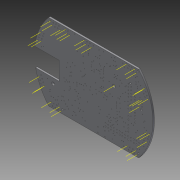
# Autodesk Inventor part: beep_main_new
Saved by Autodesk Inventor 2014 (Build 180170000, 170)
## iProperties
Created: 2013-08-27
Part Number: beep_main_new
Material: Generisch
Document SubType Name: Modeling
Designer: Felix
Density: 1 g/cm^3
Appearance: Vorgabe
Author: Felix
Autodesk Inventor part; units mm, degrees
ref_plane "YZ Plane" through (0, 0, 0) normal (1, 0, 0) x (0, 1, 0)
ref_plane "XZ Plane" through (0, 0, 0) normal (0, 1, 0) x (-1, 0, 0)
ref_plane "XY Plane" through (0, 0, 0) normal (0, 0, 1) x (1, 0, 0)
sketch "Skizze2" plane through (0, 0, 0) normal (0, 1, 0) x (-1, 0, 0)
  circle A0 centre (77.705, 71.07) radius 0.75
  circle A1 centre (17.77, 43.405) radius 0.75
  circle A2 centre (17.67, 60.315) radius 0.75
  circle A3 centre (7.87, 44.425) radius 0.75
  circle A4 centre (11.055, 72.63) radius 0.75
  circle A5 centre (10.255, 9.23) radius 0.75
  arc A6 (10.3, 74.8) -> (10.3, 5.7) centre (50.45, 40.25) ccw
  circle A7 centre (60.675, 71.27) radius 0.75
  circle A8 centre (78.855, 9.13) radius 0.75
  circle A9 centre (91.045, 71.07) radius 0.75
  circle A10 centre (32.7, 50.6) radius 1.4
  circle A11 centre (87.3, 25.1) radius 1.4
  arc A12 (91.4, 5.7) -> (103.1, 29.6999) centre (50.8775, 40.3065) ccw
  arc A13 (103.8, 46.0999) -> (91.4, 74.8) centre (50.8494, 40.2512) ccw
  line L0 (81.9, 29.6999) -> (103.1, 29.6999)
  line L1 (81.9, 46.0999) -> (81.9, 29.6999)
  line L2 (103.8, 46.0999) -> (81.9, 46.0999)
  line L3 (10.3, 5.7) -> (91.4, 5.7)
  line L4 (10.3, 74.8) -> (91.4, 74.8)
  circle A14 centre (32.9, 25.7) radius 0.254
  circle A15 centre (41.7, 37.3) radius 0.254
  circle A16 centre (44, 39.8) radius 0.254
  circle A17 centre (42, 14.1) radius 0.254
  circle A18 centre (52.4, 59.6) radius 0.254
  circle A19 centre (52.9, 55.5) radius 0.254
  circle A20 centre (52.9, 57) radius 0.254
  circle A21 centre (55.6, 64.7) radius 0.254
  circle A22 centre (54.6, 67.8) radius 0.254
  circle A23 centre (73.4, 19.4) radius 0.254
  circle A24 centre (78.1, 19.4) radius 0.254
  circle A25 centre (77.4, 16.7) radius 0.254
  circle A26 centre (70.2, 16.8) radius 0.254
  circle A27 centre (77.3, 24.7) radius 0.254
  circle A28 centre (72.9, 27.3) radius 0.254
  circle A29 centre (22.25, 50.95) radius 0.254
  circle A30 centre (30.1, 38) radius 0.254
  circle A31 centre (31.9, 59.9) radius 0.254
  circle A32 centre (27.7, 33) radius 0.254
  circle A33 centre (28.8, 43.2) radius 0.254
  circle A34 centre (30.3, 34.6) radius 0.254
  circle A35 centre (34, 41.7) radius 0.254
  circle A36 centre (32.3, 57.4) radius 0.254
  circle A37 centre (70.6, 42.4) radius 0.254
  circle A38 centre (24.5, 72.5) radius 0.254
  circle A39 centre (71.1, 39.3) radius 0.254
  circle A40 centre (11.2, 60.8) radius 0.254
  circle A41 centre (22.2, 27.1) radius 0.254
  circle A42 centre (72.3, 38.7) radius 0.254
  circle A43 centre (38.7, 23.6) radius 0.254
  circle A44 centre (76, 14.9) radius 0.254
  circle A45 centre (34, 19.5) radius 0.254
  circle A46 centre (75.2, 44) radius 0.254
  circle A47 centre (76.7, 10.1) radius 0.254
  circle A48 centre (10.5, 64.9) radius 0.254
  circle A49 centre (4.7, 37.2) radius 0.254
  circle A50 centre (92.4, 26.6) radius 0.254
  circle A51 centre (62.5, 17.2) radius 0.254
  circle A52 centre (82.8, 17.4) radius 0.254
  circle A53 centre (67.8, 12.5) radius 0.254
  circle A54 centre (37.3, 21) radius 0.254
  circle A55 centre (82.7, 11.6) radius 0.254
  circle A56 centre (8.4, 63) radius 0.254
  circle A57 centre (30, 65.2) radius 0.254
  circle A58 centre (43.5, 43.4) radius 0.254
  circle A59 centre (5.7, 35.9) radius 0.254
  circle A60 centre (9.5, 12.8) radius 0.254
  circle A61 centre (36.7, 23.3) radius 0.254
  circle A62 centre (64.6, 17.4) radius 0.254
  circle A63 centre (3.3, 30.6) radius 0.254
  circle A64 centre (69.1, 12.5) radius 0.254
  circle A65 centre (90.2, 17.7) radius 0.254
  circle A66 centre (13.1, 67.2) radius 0.254
  circle A67 centre (11.7, 68.6) radius 0.254
  circle A68 centre (31.4, 66.7) radius 0.254
  circle A69 centre (43.6, 44.9) radius 0.254
  circle A70 centre (11.5, 12.1) radius 0.254
  circle A71 centre (70, 9) radius 0.254
  circle A72 centre (35.2, 22.6) radius 0.254
  circle A73 centre (90.1, 19.2) radius 0.254
  circle A74 centre (63.5, 15.5) radius 0.254
  circle A75 centre (14.7, 68.1) radius 0.254
  circle A76 centre (30.06, 67.74) radius 0.254
  circle A77 centre (42, 45) radius 0.254
  circle A78 centre (57.4, 38.4) radius 0.254
  circle A79 centre (37, 26.4) radius 0.254
  circle A80 centre (31.4, 25.7) radius 0.254
  circle A81 centre (63.5, 21.7) radius 0.254
  circle A82 centre (11.2, 59.3) radius 0.254
  circle A83 centre (23.7, 27.1) radius 0.254
  circle A84 centre (64.7, 24.4) radius 0.254
  circle A85 centre (35.6, 24.7) radius 0.254
  circle A86 centre (30.6, 23.7) radius 0.254
  circle A87 centre (65.5, 26.3) radius 0.254
  circle A88 centre (66.6, 29.3) radius 0.254
  circle A89 centre (79.7, 15.9) radius 0.254
  circle A90 centre (67.7, 30.3) radius 0.254
  circle A91 centre (97.8, 48.7) radius 0.254
  circle A92 centre (76.6, 32) radius 0.254
  circle A93 centre (74.1, 33.1) radius 0.254
  circle A94 centre (41.9, 55.5) radius 0.254
  circle A95 centre (77.5, 34.5) radius 0.254
  circle A96 centre (32.9, 70.3) radius 0.254
  circle A97 centre (26.85, 36.1) radius 0.254
  circle A98 centre (31.7, 12.5) radius 0.254
  circle A99 centre (12.6, 63.9) radius 0.254
  circle A100 centre (67.7, 48.9) radius 0.254
  circle A101 centre (95.9, 49.8) radius 0.254
  circle A102 centre (62, 37.1) radius 0.254
  circle A103 centre (62.9, 26.4) radius 0.254
  circle A104 centre (62.4, 47.4) radius 0.254
  circle A105 centre (73.5, 12.3) radius 0.254
  circle A106 centre (48.4, 36.7) radius 0.254
  circle A107 centre (68.9, 35.1) radius 0.254
  circle A108 centre (44.6, 51) radius 0.254
  circle A109 centre (59.5, 34.2) radius 0.254
  circle A110 centre (39.1, 36.7) radius 0.254
  circle A111 centre (54.2, 36.7) radius 0.254
  circle A112 centre (51.1, 72.8) radius 0.254
  circle A113 centre (31.8, 73.1) radius 0.254
  circle A114 centre (49, 45) radius 0.254
  circle A115 centre (42.2, 49.9) radius 0.254
  circle A116 centre (66.8, 10.8) radius 0.254
  circle A117 centre (85.4, 13.4) radius 0.254
  circle A118 centre (21.8, 20.7) radius 0.254
  circle A119 centre (30.2, 36.3) radius 0.254
  circle A120 centre (41.8, 57.1) radius 0.254
  circle A121 centre (58.5, 10.5) radius 0.254
  circle A122 centre (53.7, 39.4) radius 0.254
  circle A123 centre (52, 34.2) radius 0.254
  circle A124 centre (56.4, 26.4) radius 0.3
  circle A125 centre (61.1, 11.6) radius 0.254
  circle A126 centre (26.9, 58) radius 0.254
  circle A127 centre (6.5, 19.3) radius 0.254
  circle A128 centre (17.1, 34.8) radius 0.254
  circle A129 centre (5.7, 26.7) radius 0.254
  circle A130 centre (5.6, 16.8) radius 0.254
  circle A131 centre (34, 8.5) radius 0.254
  circle A132 centre (41.8, 58.5) radius 0.254
  circle A133 centre (45.1, 53.9) radius 0.254
  circle A134 centre (50.3, 54.3) radius 0.254
  circle A135 centre (67.9, 73.5) radius 0.254
  circle A136 centre (47.2, 65.3) radius 0.254
  circle A137 centre (46, 72.1) radius 0.254
  circle A138 centre (41, 61.6) radius 0.3
  circle A139 centre (42, 72.7) radius 0.254
  circle A140 centre (32.9, 66.6) radius 0.254
  circle A141 centre (44.9, 43.2) radius 0.254
  circle A142 centre (29.6, 29.9) radius 0.254
  circle A143 centre (16.7, 29.4) radius 0.254
  circle A144 centre (12.7, 24.2) radius 0.254
  circle A145 centre (65.9, 35.5) radius 0.254
  circle A146 centre (61.3, 43.4) radius 0.254
  circle A147 centre (72.1, 30.3) radius 0.254
  circle A148 centre (59, 51) radius 0.254
  circle A149 centre (58.4, 46.9) radius 0.254
  circle A150 centre (79.4, 19.3) radius 0.254
  circle A151 centre (65.9, 36.9) radius 0.254
  circle A152 centre (45.2, 68.1) radius 0.254
  circle A153 centre (34.6, 72) radius 0.254
  circle A154 centre (29.2, 60.5) radius 0.254
  circle A155 centre (36.7, 64) radius 0.254
  circle A156 centre (44.5, 60.4) radius 0.254
  circle A157 centre (12.6, 62.1) radius 0.254
  circle A158 centre (38.9, 64.9) radius 0.254
  circle A159 centre (22.4, 55.2) radius 0.254
  circle A160 centre (15.1, 28.8) radius 0.254
  circle A161 centre (45.6, 61.4) radius 0.254
  circle A162 centre (45.6, 65.5) radius 0.254
  circle A163 centre (25.4, 56.5) radius 0.254
  circle A164 centre (35.5, 64.8) radius 0.254
  circle A165 centre (29.3, 22.4) radius 0.254
  circle A166 centre (25.4, 11.6) radius 0.254
  circle A167 centre (58.5, 39.5) radius 0.3
  circle A168 centre (45.3, 55.9) radius 0.254
  circle A169 centre (64.5, 28.9) radius 0.254
  circle A170 centre (86.9, 14.5) radius 0.254
  circle A171 centre (46.7, 55.9) radius 0.254
  circle A172 centre (71.9, 41.7) radius 0.254
  circle A173 centre (48.2, 55.8) radius 0.254
  circle A174 centre (70, 50.1) radius 0.254
  circle A175 centre (71.8, 46.1) radius 0.254
  circle A176 centre (50.8, 61.1) radius 0.254
  circle A177 centre (59.9, 37.2) radius 0.254
  circle A178 centre (6.8, 41.4) radius 0.254
  circle A179 centre (11.3, 26.4) radius 0.254
  circle A180 centre (55.7, 66.7) radius 0.254
  circle A181 centre (45.8, 22.8) radius 0.254
  circle A182 centre (44.9, 26) radius 0.254
  circle A183 centre (72.5, 33.9) radius 0.254
  circle A184 centre (34.6, 31.6) radius 0.254
  circle A185 centre (23.5, 23.3) radius 0.254
  circle A186 centre (21.5, 56.3) radius 0.254
  circle A187 centre (9.1, 53.3) radius 0.254
  circle A188 centre (74.2, 47.9) radius 0.254
  circle A189 centre (75.5, 33.9) radius 0.254
  circle A190 centre (60.3, 17.1) radius 0.254
  circle A191 centre (35.9, 20.5) radius 0.254
  circle A192 centre (32.7, 20.5) radius 0.254
  circle A193 centre (89.105, 14.395) radius 0.254
  circle A194 centre (83.6, 14.3) radius 0.254
  circle A195 centre (74.7, 13.7) radius 0.254
  circle A196 centre (23.9, 8) radius 0.254
  circle A197 centre (23.9, 11.6) radius 0.254
  circle A198 centre (5.2, 31.8) radius 0.254
  circle A199 centre (10.4, 20.5) radius 0.254
  circle A200 centre (23.03, 70.23) radius 0.254
  circle A201 centre (41.7, 53) radius 0.254
  circle A202 centre (43.2, 51.5) radius 0.254
  circle A203 centre (44.1, 57.8) radius 0.254
  circle A204 centre (31.4, 70.3) radius 0.254
  circle A205 centre (40.4, 42.8) radius 0.254
  circle A206 centre (22.7, 43.5) radius 0.254
  circle A207 centre (19.9, 45) radius 0.254
  circle A208 centre (58.2, 64.5) radius 0.254
  circle A209 centre (65.6, 61.3) radius 0.254
  circle A210 centre (55.6, 63.3) radius 0.254
  circle A211 centre (46.2, 27.8) radius 0.254
  circle A212 centre (61, 69.2) radius 0.254
  circle A213 centre (50.4, 52.8) radius 0.254
  circle A214 centre (52.5, 52.8) radius 0.254
  circle A215 centre (41.8, 60) radius 0.254
  circle A216 centre (48.8, 39.9) radius 0.254
  circle A217 centre (45.9, 39.8) radius 0.254
  circle A218 centre (30.1, 39.4) radius 0.254
  circle A219 centre (37.1, 13.3) radius 0.254
  circle A220 centre (33.2, 13.3) radius 0.254
  circle A221 centre (76.305, 72.87) radius 0.4064
  circle A222 centre (75.035, 70.33) radius 0.4064
  circle A223 centre (73.765, 72.87) radius 0.4064
  circle A224 centre (72.495, 70.33) radius 0.4064
  circle A225 centre (60.3, 44.5) radius 0.254
  circle A226 centre (19.57, 42.005) radius 0.4064
  circle A227 centre (17.03, 40.735) radius 0.4064
  circle A228 centre (19.57, 39.465) radius 0.4064
  circle A229 centre (17.03, 38.195) radius 0.4064
  circle A230 centre (65.9, 33.9) radius 0.254
  circle A231 centre (19.47, 58.915) radius 0.4064
  circle A232 centre (16.93, 57.645) radius 0.4064
  circle A233 centre (19.47, 56.375) radius 0.4064
  circle A234 centre (16.93, 55.105) radius 0.4064
  circle A235 centre (19.47, 53.835) radius 0.4064
  circle A236 centre (16.93, 52.565) radius 0.4064
  circle A237 centre (19.47, 51.295) radius 0.4064
  circle A238 centre (16.93, 50.025) radius 0.4064
  circle A239 centre (19.47, 48.755) radius 0.4064
  circle A240 centre (16.93, 47.485) radius 0.4064
  circle A241 centre (71.9, 28.8) radius 0.254
  circle A242 centre (9.67, 45.825) radius 0.4064
  circle A243 centre (7.13, 47.095) radius 0.4064
  circle A244 centre (9.67, 48.365) radius 0.4064
  circle A245 centre (7.13, 49.635) radius 0.4064
  circle A246 centre (9.67, 50.905) radius 0.4064
  circle A247 centre (7.13, 52.175) radius 0.4064
  circle A248 centre (63.4, 37) radius 0.254
  circle A249 centre (12.455, 70.83) radius 0.4064
  circle A250 centre (13.725, 73.37) radius 0.4064
  circle A251 centre (14.995, 70.83) radius 0.4064
  circle A252 centre (16.265, 73.37) radius 0.4064
  circle A253 centre (17.535, 70.83) radius 0.4064
  circle A254 centre (18.805, 73.37) radius 0.4064
  circle A255 centre (20.075, 70.83) radius 0.4064
  circle A256 centre (21.345, 73.37) radius 0.4064
  circle A257 centre (59.2, 45.4) radius 0.254
  circle A258 centre (11.655, 7.43) radius 0.4064
  circle A259 centre (12.925, 9.97) radius 0.4064
  circle A260 centre (14.195, 7.43) radius 0.4064
  circle A261 centre (15.465, 9.97) radius 0.4064
  circle A262 centre (16.735, 7.43) radius 0.4064
  circle A263 centre (18.005, 9.97) radius 0.4064
  circle A264 centre (19.275, 7.43) radius 0.4064
  circle A265 centre (20.545, 9.97) radius 0.4064
  circle A266 centre (67.5, 21.8) radius 0.254
  circle A267 centre (4.9078, 62.6827) radius 0.4064
  circle A268 centre (6.7307, 60.5053) radius 0.4064
  circle A269 centre (3.895, 60.3534) radius 0.4064
  circle A270 centre (5.7179, 58.1759) radius 0.4064
  circle A271 centre (2.8821, 58.0241) radius 0.4064
  circle A272 centre (4.705, 55.8466) radius 0.4064
  circle A273 centre (1.8693, 55.6947) radius 0.4064
  circle A274 centre (3.6922, 53.5173) radius 0.4064
  circle A275 centre (0.3852, 29.2123) radius 0.4064
  circle A276 centre (3.1969, 28.8139) radius 0.4064
  circle A277 centre (1.1912, 26.8036) radius 0.4064
  circle A278 centre (4.0029, 26.4052) radius 0.4064
  circle A279 centre (1.9971, 24.3948) radius 0.4064
  circle A280 centre (4.8088, 23.9964) radius 0.4064
  circle A281 centre (2.8031, 21.9861) radius 0.4064
  circle A282 centre (5.6148, 21.5877) radius 0.4064
  circle A283 centre (59.275, 73.07) radius 0.4064
  circle A284 centre (58.005, 70.53) radius 0.4064
  circle A285 centre (56.735, 73.07) radius 0.4064
  circle A286 centre (55.465, 70.53) radius 0.4064
  circle A287 centre (54.195, 73.07) radius 0.4064
  circle A288 centre (30, 57.6) radius 0.254
  circle A289 centre (24.5, 48.9) radius 0.254
  circle A290 centre (80.255, 7.33) radius 0.4064
  circle A291 centre (81.525, 9.87) radius 0.4064
  circle A292 centre (82.795, 7.33) radius 0.4064
  circle A293 centre (84.065, 9.87) radius 0.4064
  circle A294 centre (85.335, 7.33) radius 0.4064
  circle A295 centre (86.605, 9.87) radius 0.4064
  circle A296 centre (87.875, 7.33) radius 0.4064
  circle A297 centre (89.145, 9.87) radius 0.4064
  circle A298 centre (30.9, 58.9) radius 0.254
  circle A299 centre (89.645, 72.87) radius 0.4064
  circle A300 centre (88.375, 70.33) radius 0.4064
  circle A301 centre (87.105, 72.87) radius 0.4064
  circle A302 centre (85.835, 70.33) radius 0.4064
  circle A303 centre (84.565, 72.87) radius 0.4064
  circle A304 centre (83.295, 70.33) radius 0.4064
  circle A305 centre (82.025, 72.87) radius 0.4064
  circle A306 centre (80.755, 70.33) radius 0.4064
  circle A307 centre (26.6, 45.4) radius 0.254
  circle A308 centre (97.1044, 17.2038) radius 0.4064
  circle A309 centre (95.2288, 19.3361) radius 0.4064
  circle A310 centre (98.06, 19.5572) radius 0.4064
  circle A311 centre (96.1844, 21.6895) radius 0.4064
  circle A312 centre (99.0156, 21.9105) radius 0.4064
  circle A313 centre (97.14, 24.0428) radius 0.4064
  circle A314 centre (99.9712, 24.2639) radius 0.4064
  circle A315 centre (98.0956, 26.3962) radius 0.4064
  circle A316 centre (101.1281, 52.2968) radius 0.4064
  circle A317 centre (98.315, 52.6854) radius 0.4064
  circle A318 centre (100.3137, 54.7027) radius 0.4064
  circle A319 centre (97.5006, 55.0913) radius 0.4064
  circle A320 centre (99.4994, 57.1087) radius 0.4064
  circle A321 centre (96.6863, 57.4973) radius 0.4064
  circle A322 centre (98.685, 59.5146) radius 0.4064
  circle A323 centre (95.8719, 59.9032) radius 0.4064
  circle A324 centre (27.6, 53.1) radius 0.254
  circle A325 centre (27.4, 43.2) radius 0.254
  circle A326 centre (40.6488, 11.4606) radius 0.508
  circle A327 centre (47.1512, 11.4606) radius 0.508
  circle A328 centre (40.6488, 6.9394) radius 0.508
  circle A329 centre (47.1512, 6.9394) radius 0.508
  circle A330 centre (60.1, 54.96) radius 0.4064
  circle A331 centre (60.1, 60.04) radius 0.4064
  circle A332 centre (19.43, 33.62) radius 0.508
  circle A333 centre (19.43, 31.08) radius 0.508
  circle A334 centre (19.47, 21.59) radius 0.508
  circle A335 centre (19.47, 24.13) radius 0.508
  circle A336 centre (52.925, 70.53) radius 0.4064
  circle A337 centre (35.032, 15.304) radius 0.508
  circle A338 centre (29.952, 15.304) radius 0.508
  circle A339 centre (27.412, 15.304) radius 0.508
  circle A340 centre (27.412, 17.844) radius 0.508
  circle A341 centre (24.872, 17.844) radius 0.508
  circle A342 centre (22.332, 15.304) radius 0.508
  circle A343 centre (22.332, 17.844) radius 0.508
  circle A344 centre (19.792, 15.304) radius 0.508
  circle A345 centre (17.252, 15.304) radius 0.508
  circle A346 centre (37.572, 17.844) radius 0.508
  circle A347 centre (32.492, 17.844) radius 0.508
  circle A348 centre (35.032, 17.844) radius 0.508
  circle A349 centre (37.572, 15.304) radius 0.508
  circle A350 centre (40.112, 15.304) radius 0.508
  circle A351 centre (17.252, 17.844) radius 0.508
  circle A352 centre (14.712, 17.844) radius 0.508
  circle A353 centre (12.172, 17.844) radius 0.508
  circle A354 centre (32.492, 15.304) radius 0.508
  circle A355 centre (24.872, 15.304) radius 0.508
  circle A356 centre (14.712, 15.304) radius 0.508
  circle A357 centre (40.112, 17.844) radius 0.508
  circle A358 centre (19.792, 17.844) radius 0.508
  circle A359 centre (12.172, 15.304) radius 0.508
  circle A360 centre (9.632, 15.304) radius 0.508
  circle A361 centre (29.952, 17.844) radius 0.508
  circle A362 centre (9.632, 17.844) radius 0.508
  circle A363 centre (13.4, 54.57) radius 0.508
  circle A364 centre (13.4, 44.41) radius 0.508
  circle A365 centre (13.4, 46.95) radius 0.508
  circle A366 centre (13.4, 34.25) radius 0.508
  circle A367 centre (13.4, 31.71) radius 0.508
  circle A368 centre (13.4, 41.87) radius 0.508
  circle A369 centre (13.4, 36.79) radius 0.508
  circle A370 centre (13.4, 49.49) radius 0.508
  circle A371 centre (13.4, 39.33) radius 0.508
  circle A372 centre (13.4, 52.03) radius 0.508
  circle A373 centre (38.684, 39.4) radius 0.4064
  circle A374 centre (40.716, 39.4) radius 0.4064
  circle A375 centre (25.084, 29.4) radius 0.4064
  circle A376 centre (27.116, 29.4) radius 0.4064
  circle A377 centre (27, 40) radius 0.254
  circle A378 centre (29.2, 25.3) radius 0.254
  circle A379 centre (36.9, 52.1) radius 0.254
  circle A380 centre (36, 42.7) radius 0.254
  circle A381 centre (29.7, 32.3) radius 0.254
  circle A382 centre (29.8, 27.1) radius 0.254
  circle A383 centre (49, 65.4) radius 0.254
  circle A384 centre (19.47, 26.67) radius 0.508
  point P0 (0, 0)
  constraints: 385 centre point, 10 end point, 8 point on circle
extrude "Extrusion1" add sketch "Skizze2" along normal blind 1.5
